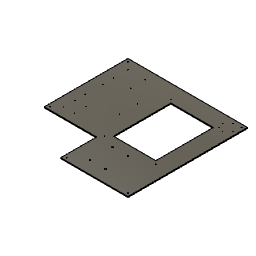
5780 Board v1 (Autodesk Fusion 360 design; units mm, degrees)
Autodesk Fusion 360 part; units mm, degrees
sketch "Sketch1" plane through (0, 0, 0) normal (0, 0, 1) x (1, 0, 0)
  line L0 (-100, 50) -> (300, 50)
  line L1 (300, 50) -> (300, -350)
  line L2 (300, -350) -> (-100, -350)
  line L3 (-100, -350) -> (-100, 50)
  dimension "d1" = 400
  dimension "d2" = 400
  constraint horizontal L0
  constraint vertical L1
  constraint horizontal L2
  constraint vertical L3
  measures "d1" distance of L0.start L0.end
  measures "d2" distance of L0.start L2.end
extrude "Extrude1" add sketch "Sketch1" along normal blind 3
sketch "Sketch2" plane through (0, 0, 3) normal (0, 0, 1) x (-1, 0, 0)
  line L0 (100, 350) -> (-300, 350)
  line L1 (-300, 350) -> (-300, -50)
  line L2 (-300, -50) -> (100, -50)
  line L3 (100, -50) -> (100, 350)
  line L4 (-263.3486, -40) -> (-290, -13.1239)
  line L5 (-290, -13.1239) -> (-270.7994, 7.2868)
  line L6 (-270.7994, 7.2868) -> (-243.7577, -19.9951)
  line L7 (-243.7577, -19.9951) -> (-263.3486, -40)
  circle A0 centre (-263.3392, -37.3821) radius 1
  circle A1 centre (-287.4151, -13.0924) radius 1
  circle A2 centre (-246.3371, -20.0207) radius 1
  circle A3 centre (-270.413, 4.269) radius 1
  line L8 (-105, 220) -> (-270, 220)
  line L9 (-270, 220) -> (-270, 320)
  line L10 (-270, 320) -> (-105, 320)
  line L11 (-105, 320) -> (-105, 220)
  circle A4 centre (-130.5, 232.5) radius 2.5
  circle A5 centre (-130.5, 307.5) radius 2.5
  circle A6 centre (-182.5, 232.5) radius 2.5
  circle A7 centre (-182.5, 307.5) radius 2.5
  line L12 (-152.9998, 228.0039) -> (-160.7739, 228.0044) construction
  line L13 (-160.7739, 228.0044) -> (-160.7741, 225.0005) construction
  line L14 (-160.7741, 225.0005) -> (-153, 225) construction
  line L15 (-153, 225) -> (-152.9998, 228.0039) construction
  line L16 (-153, 315) -> (-168.7144, 314.9704) construction
  line L17 (-168.7144, 314.9704) -> (-168.6983, 306.4348) construction
  line L18 (-168.6983, 306.4348) -> (-152.9839, 306.4644) construction
  line L19 (-152.9839, 306.4644) -> (-153, 315) construction
  line L20 (-49.76, 127.68) -> (70, 127.68)
  circle A8 centre (67.5, 66.3) radius 1.25
  line L21 (70, 127.68) -> (70, 63.8)
  circle A9 centre (-47.26, 125.18) radius 1.25
  circle A10 centre (67.5, 125.18) radius 1.25
  line L22 (-49.76, 63.8) -> (-49.76, 127.68)
  circle A11 centre (-47.26, 66.3) radius 1.25
  line L23 (70, 63.8) -> (-49.76, 63.8)
  line L24 (70, -20) -> (6.9, -20)
  line L25 (70, 33.8) -> (70, -20)
  line L26 (6.9, -20) -> (6.9, 33.8)
  circle A12 centre (9.4, 31.3) radius 1.25
  circle A13 centre (9.4, -17.5) radius 1.25
  circle A14 centre (67.5, 31.3) radius 1.25
  circle A15 centre (67.5, -17.5) radius 1.25
  line L27 (6.9, 33.8) -> (70, 33.8)
  circle A16 centre (67.5, 197.68) radius 1.25
  line L28 (70, 157.68) -> (28.7, 157.68)
  circle A17 centre (67.5, 160.18) radius 1.25
  line L29 (70, 200.18) -> (70, 157.68)
  circle A18 centre (31.2, 197.68) radius 1.25
  line L30 (28.7, 200.18) -> (70, 200.18)
  line L31 (28.7, 157.68) -> (28.7, 200.18)
  circle A19 centre (31.2, 160.18) radius 1.25
  dimension "d5" = 2
  dimension "d6" = 2
  dimension "d7" = 2
  dimension "d8" = 2
  dimension "d9" = 34.2
  dimension "d10" = 24.3
  dimension "d11" = 34.2
  dimension "d12" = 24.3
  dimension "d13" = 37.85
  dimension "d14" = 28
  dimension "d15" = 1.85
  dimension "d16" = 1.85
  dimension "d17" = 1.85
  dimension "d18" = 1.825
  dimension "d19" = 1.825
  dimension "d20" = 100
  dimension "d21" = 165
  dimension "d22" = 5
  dimension "d23" = 5
  dimension "d24" = 5
  dimension "d25" = 5
  dimension "d26" = 52
  dimension "d27" = 75
  dimension "d28" = 52
  dimension "d29" = 75
  dimension "d30" = 25.5
  dimension "d31" = 25.5
  dimension "d32" = 12.5
  dimension "d33" = 10
  dimension "d34" = 10
  dimension "d35" = 87.5
  dimension "d36" = 12.5
  dimension "d37" = 5
  dimension "d38" = 48
  dimension "d39" = 5
  dimension "d40" = 48
  dimension "d190" = 10
  dimension "d42" = 2.5
  dimension "d43" = 2.5
  dimension "d44" = 2.5
  dimension "d45" = 2.5
  dimension "d46" = 2.5
  dimension "d47" = 2.5
  dimension "d48" = 2.5
  dimension "d49" = 2.5
  dimension "d50" = 2.5
  dimension "d51" = 2.5
  dimension "d52" = 2.5
  dimension "d53" = 114.76
  dimension "d54" = 58.88
  dimension "d55" = 58.88
  dimension "d56" = 2.5
  dimension "d57" = 114.76
  dimension "d186" = 10
  dimension "d59" = 2.5
  dimension "d60" = 2.5
  dimension "d61" = 2.5
  dimension "d62" = 2.5
  dimension "d63" = 2.5
  dimension "d64" = 2.5
  dimension "d65" = 2.5
  dimension "d66" = 2.5
  dimension "d67" = 2.5
  dimension "d68" = 2.5
  dimension "d69" = 2.5
  dimension "d70" = 58.1
  dimension "d71" = 48.8
  dimension "d72" = 48.8
  dimension "d188" = 10
  dimension "d74" = 2.5
  dimension "d75" = 2.5
  dimension "d76" = 2.5
  dimension "d77" = 2.5
  dimension "d78" = 2.5
  dimension "d79" = 2.5
  dimension "d80" = 2.5
  dimension "d81" = 2.5
  dimension "d82" = 2.5
  dimension "d83" = 2.5
  dimension "d84" = 2.5
  dimension "d85" = 37.5
  dimension "d86" = 36.3
  dimension "d87" = 36.3
  dimension "d90" = 30
  dimension "d91" = 58.1
  dimension "d92" = 30
  dimension "d93" = 30
  dimension "d94" = 30
  dimension "d95" = 30
  dimension "d96" = 30
  dimension "d97" = 12.5
  dimension "d98" = 87.5
  dimension "d99" = 10
  dimension "d100" = 10
  dimension "d101" = 30
  dimension "d102" = 30
  constraint horizontal L28
  constraint vertical L31
  constraint horizontal L30
  constraint vertical L29
  measures "d5" diameter of A0
  measures "d6" diameter of A1
  measures "d7" diameter of A2
  measures "d8" diameter of A3
  measures "d9" distance of A0.centre A1.centre
  measures "d10" distance of A0.centre A2.centre
  measures "d11" distance of A2.centre A3.centre
  measures "d12" distance of A1.centre A3.centre
  measures "d13" distance of L4.start L4.end
  measures "d14" distance of L4.start L6.end
  measures "d15" distance of L4 A0.centre
  measures "d16" distance of L6 A2.centre
  measures "d17" distance of L6 A3.centre
  measures "d18" distance of L7 A0.centre
  measures "d19" distance of L7 A2.centre
  measures "d20" distance of L8.start L10.end
  measures "d21" distance of L8.start L8.end
  measures "d22" diameter of A4
  measures "d23" diameter of A5
  measures "d24" diameter of A6
  measures "d25" diameter of A7
  measures "d26" distance of A4.centre A6.centre
  measures "d27" distance of A4.centre A5.centre
  measures "d28" distance of A5.centre A7.centre
  measures "d29" distance of A6.centre A7.centre
  measures "d30" distance of L11 A4.centre
  measures "d31" distance of L11 A5.centre
  measures "d32" distance of L8 A4.centre
  measures "d35" distance of L9 A6.centre
  measures "d36" distance of L8 A6.centre
  measures "d42" diameter of A11
  measures "d43" diameter of A8
  measures "d44" diameter of A10
  measures "d45" distance of A11.centre L22
  measures "d46" distance of A11.centre L23
  measures "d47" diameter of A9
  measures "d48" distance of A9.centre L22
  measures "d49" distance of A9.centre L20
  measures "d50" distance of A8.centre L23
  measures "d51" distance of A8.centre L21
  measures "d52" distance of A10.centre L21
  measures "d53" distance of A11.centre A8.centre
  measures "d54" distance of A11.centre A9.centre
  measures "d55" distance of A8.centre A10.centre
  measures "d56" distance of A10.centre L20
  measures "d57" distance of A9.centre A10.centre
  measures "d59" diameter of A14
  measures "d60" diameter of A12
  measures "d61" diameter of A13
  measures "d62" distance of A14.centre L25
  measures "d63" distance of A14.centre L27
  measures "d64" diameter of A15
  measures "d65" distance of A15.centre L25
  measures "d66" distance of A15.centre L24
  measures "d67" distance of A12.centre L27
  measures "d68" distance of A12.centre L26
  measures "d69" distance of A13.centre L26
  measures "d70" distance of A14.centre A12.centre
  measures "d71" distance of A14.centre A15.centre
  measures "d72" distance of A13.centre A12.centre
  measures "d74" diameter of A17
  measures "d75" diameter of A16
  measures "d76" diameter of A18
  measures "d77" distance of A17.centre L28
  measures "d78" distance of A17.centre L29
  measures "d79" diameter of A19
  measures "d80" distance of A19.centre L28
  measures "d81" distance of A19.centre L31
  measures "d82" distance of A16.centre L29
  measures "d83" distance of A16.centre L30
  measures "d84" distance of A18.centre L30
  measures "d85" distance of A17.centre A16.centre
  measures "d86" distance of A17.centre A19.centre
  measures "d87" distance of A16.centre A18.centre
  measures "d90" distance of L3 L25
  measures "d91" distance of A13.centre A15.centre
  measures "d92" distance of L2 L24
  measures "d93" distance of L23 L27
  measures "d94" distance of L20 L28
  measures "d95" distance of L3 L29
  measures "d96" distance of L3 L21
  measures "d97" distance of L10 A7.centre
  measures "d98" distance of L9 A7.centre
  measures "d99" distance of L1 L4.end
  measures "d100" distance of L2 L4.start
  measures "d101" distance of L1 L9
  measures "d102" distance of L0 L10
sketch "Sketch3" plane through (0, 0, 3) normal (0, 0, 1) x (1, 0, 0)
  line L0 (-100, -350.18) -> (75, -350.18)
  line L1 (75, -350.18) -> (75, -230.18)
  line L2 (75, -230.18) -> (-100, -230.18)
  line L3 (-100, -230.18) -> (-100, -350.18)
  line L4 (-28.7, -200.18) -> (-70, -200.18)
  line L5 (105, -320) -> (105, -220)
  dimension "d103" = 30
  dimension "d104" = 30
  dimension "d105" = 120
  dimension "d106" = 175
  constraint horizontal L0
  constraint vertical L1
  constraint horizontal L2
  constraint vertical L3
  measures "d103" distance of L2 L4
  measures "d104" distance of L1 L5
  measures "d105" distance of L0 L2
  measures "d106" distance of L0.start L0.end
extrude "Extrude2" cut sketch "Sketch3" against normal blind 5.5
extrude "Extrude3" cut sketch "Sketch2" against normal blind 5.5 contours A4 | A5 | A6 | A7 | A8 | A9 | A10 | A11 | A12 | A13 | A14 | A15 | A16 | A17 | A18 | A19
extrude "Extrude4" cut sketch "Sketch2" against normal blind 5.5 contours A0 | A1 | A2 | A3
sketch "Sketch4" plane through (0, 0, 3) normal (0, 0, 1) x (-1, 0, 0)
  circle A0 centre (-270.413, 4.269) radius 1
  circle A1 centre (-287.4151, -13.0924) radius 1
  circle A2 centre (-246.3371, -20.0207) radius 1
  circle A3 centre (-263.3392, -37.3821) radius 1
  circle A4 centre (9.4, 31.3) radius 1.25
  circle A5 centre (-47.26, 125.18) radius 1.25
  circle A6 centre (31.2, 160.18) radius 1.25
  circle A7 centre (-130.5, 232.5) radius 2.5
  circle A8 centre (-182.5, 307.5) radius 2.5
  circle A9 centre (67.5, 197.68) radius 1.25
  circle A10 centre (-47.26, 66.3) radius 1.25
  circle A11 centre (9.4, -17.5) radius 1.25
  circle A12 centre (67.5, 31.3) radius 1.25
  circle A13 centre (67.5, 125.18) radius 1.25
  circle A14 centre (31.2, 197.68) radius 1.25
  circle A15 centre (-130.5, 307.5) radius 2.5
  circle A16 centre (-182.5, 232.5) radius 2.5
  circle A17 centre (67.5, 160.18) radius 1.25
  circle A18 centre (67.5, 66.3) radius 1.25
  circle A19 centre (67.5, -17.5) radius 1.25
  line L0 (-75, 230.18) -> (-75, 350)
  line L1 (-75, 350) -> (-300, 350)
  line L2 (-300, 350) -> (-300, -50)
  line L3 (-300, -50) -> (100, -50)
  line L4 (100, -50) -> (100, 230.18)
  line L5 (100, 230.18) -> (-75, 230.18)
  line L6 (-242.6879, 7.3358) -> (-100.7815, 7.3358)
  line L7 (-100.7815, 7.3358) -> (-100.7815, 199.5971)
  line L8 (-100.7815, 199.5971) -> (-242.6879, 199.5971)
  line L9 (-242.6879, 199.5971) -> (-242.6879, 7.3358)
  line L10 (-270.7994, 7.2868) -> (-243.7577, -19.9951)
  dimension "d113" = 20
  dimension "d114" = 40
  constraint horizontal L6
  constraint vertical L7
  constraint horizontal L8
  constraint vertical L9
  measures "d113" distance of L6.start L10
  measures "d114" distance of L0.start L7.end
extrude "Extrude5" cut sketch "Sketch4" against normal blind 3 contours L6 L7 L8 L9
sketch "Sketch5" plane through (0, 0, 3) normal (0, 0, 1) x (1, 0, 0)
  circle A0 centre (-90, 40) radius 1.5
  line L0 (-100, 50) -> (300, 50)
  line L1 (-100, -350) -> (-100, 50)
  circle A1 centre (290, 40) radius 1.5
  line L2 (300, 50) -> (300, -350)
  circle A2 centre (290, -340) radius 1.5
  line L3 (300, -350) -> (-100, -350)
  circle A3 centre (85, -340) radius 1.5
  line L4 (75, -230.18) -> (75, -350)
  circle A4 centre (-90, -220.18) radius 1.5
  line L5 (-100, -230.18) -> (75, -230.18)
  circle A5 centre (90.7815, 2.6642) radius 1.5
  line L6 (100.7815, -199.5971) -> (100.7815, -7.3358)
  line L7 (100.7815, -7.3358) -> (242.6879, -7.3358)
  circle A6 centre (252.6879, 2.6642) radius 1.5
  line L8 (242.6879, -7.3358) -> (242.6879, -199.5971)
  circle A7 centre (252.6879, -209.5971) radius 1.5
  line L9 (242.6879, -199.5971) -> (100.7815, -199.5971)
  circle A8 centre (85.7815, -214.5971) radius 1.5
  dimension "d117" = 3
  dimension "d118" = 10
  dimension "d119" = 10
  dimension "d120" = 3
  dimension "d121" = 10
  dimension "d122" = 10
  dimension "d123" = 3
  dimension "d124" = 10
  dimension "d125" = 10
  dimension "d126" = 3
  dimension "d127" = 10
  dimension "d128" = 10
  dimension "d129" = 3
  dimension "d130" = 10
  dimension "d131" = 10
  dimension "d132" = 3
  dimension "d133" = 10
  dimension "d134" = 10
  dimension "d135" = 3
  dimension "d136" = 10
  dimension "d137" = 10
  dimension "d138" = 3
  dimension "d139" = 10
  dimension "d140" = 10
  dimension "d141" = 3
  dimension "d142" = 15
  dimension "d143" = 15
  measures "d117" diameter of A0
  measures "d118" distance of A0.centre L0
  measures "d119" distance of A0.centre L1
  measures "d120" diameter of A1
  measures "d121" distance of L0 A1.centre
  measures "d122" distance of A1.centre L2
  measures "d123" diameter of A2
  measures "d124" distance of L2 A2.centre
  measures "d125" distance of A2.centre L3
  measures "d126" diameter of A3
  measures "d127" distance of A3.centre L4
  measures "d128" distance of L3 A3.centre
  measures "d129" diameter of A4
  measures "d130" distance of L1 A4.centre
  measures "d131" distance of A4.centre L5
  measures "d132" diameter of A5
  measures "d133" distance of A5.centre L6
  measures "d134" distance of A5.centre L7
  measures "d135" diameter of A6
  measures "d136" distance of L7 A6.centre
  measures "d137" distance of A6.centre L8
  measures "d138" diameter of A7
  measures "d139" distance of L8 A7.centre
  measures "d140" distance of A7.centre L9
  measures "d141" diameter of A8
  measures "d142" distance of L6 A8.centre
  measures "d143" distance of L9 A8.centre
extrude "Extrude6" cut sketch "Sketch5" against normal blind 3 contours A0 | A1 | A2 | A3 | A4 | A5 | A6 | A7 | A8
equation "d29 = d27"
